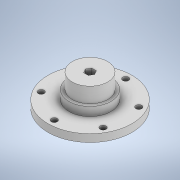
# Autodesk Inventor part: Wheel Mount
Saved by Autodesk Inventor 2020.2 (Build 242310000, 310)
## iProperties
Created: 2020-01-14
Part Number: Wheel Mount
Material: Generic
Document SubType Name: Modeling
Designer: maple
Density: 1 g/cm^3
Appearance: Default
Author: maple
Autodesk Inventor part; units mm, degrees
ref_plane "YZ Plane" through (0, 0, 0) normal (1, 0, 0) x (0, 1, 0)
ref_plane "XZ Plane" through (0, 0, 0) normal (0, 1, 0) x (-1, 0, 0)
ref_plane "XY Plane" through (0, 0, 0) normal (0, 0, 1) x (1, 0, 0)
sketch "Sketch1" plane through (0, 0, 0) normal (0, 1, 0) x (-1, 0, 0)
  circle A0 centre (0, 0) radius 27.94
  dimension "d0" = 55.88
  constraints: 1 centre point, 1 coincident
  measures "d0" diameter of A0
extrude "Extrusion1" add sketch "Sketch1" along normal blind 5.08
sketch "Sketch2" plane through (0, 5.08, 0) normal (0, 1, 0) x (1, 0, 0)
  circle A0 centre (0, 0) radius 13.97
  dimension "d3" = 27.94
  constraints: 1 centre point, 1 coincident
  measures "d3" diameter of A0
extrude "Extrusion2" add sketch "Sketch2" along normal blind 5.842
sketch "Sketch3" plane through (0, 10.922, 0) normal (0, 1, 0) x (1, 0, 0)
  circle A0 centre (0, 0) radius 11.811
  dimension "d6" = 23.622
  constraints: 1 centre point, 1 coincident
  measures "d6" diameter of A0
extrude "Extrusion3" add sketch "Sketch3" along normal blind 10.16
sketch "Sketch5" plane through (0, 21.082, 0) normal (0, 1, 0) x (1, 0, 0)
  line L0 (0, 0) -> (0, 2.667)
  line L1 (-3.1168, 0) -> (-1.5584, 2.6992)
  line L2 (-1.5584, 2.6992) -> (1.5584, 2.6992)
  line L3 (1.5584, 2.6992) -> (3.1168, 0)
  line L4 (3.1168, 0) -> (1.5584, -2.6992)
  line L5 (1.5584, -2.6992) -> (-1.5584, -2.6992)
  line L6 (-1.5584, -2.6992) -> (-3.1168, 0)
  dimension "d10" = 2.667
  constraints: 14 end point, 1 coincident, 1 vertical, 13 other
  measures "d10" distance of L0.start L0.end
extrude "Extrusion4" cut sketch "Sketch5" against normal blind 25.4
sketch "Sketch6" plane through (0, 5.08, 0) normal (0, 1, 0) x (1, 0, 0)
  circle A0 centre (0, 0) radius 27.94 projected
  circle A1 centre (0, 23.8125) radius 1.9939
  circle A2 centre (20.6222, 11.9063) radius 1.9939
  circle A3 centre (20.6222, -11.9063) radius 1.9939
  circle A4 centre (0, -23.8125) radius 1.9939
  circle A5 centre (-20.6222, -11.9063) radius 1.9939
  circle A6 centre (-20.6222, 11.9063) radius 1.9939
  constraints: 6 centre point
extrude "Extrusion5" cut sketch "Sketch6" against normal blind 25.4 contours A1 | A2 | A3 | A4 | A5 | A6
body "Solid1"
